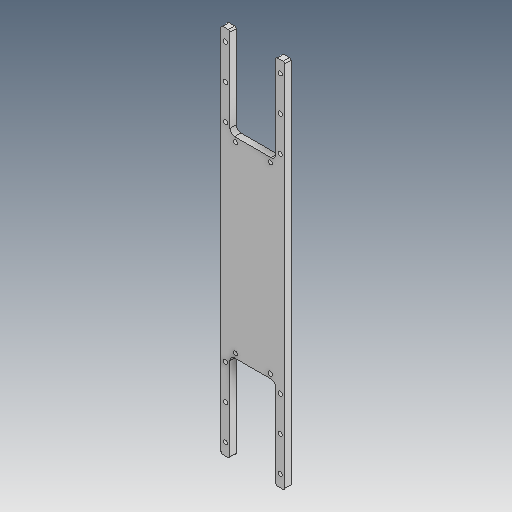
# Autodesk Inventor part: bar1
Saved by Autodesk Inventor 2020 (Build 240168000, 168)
## iProperties
Created: 2020-11-05
Part Number: bar1
Material: 일반
Document SubType Name: Sheet Metal
Designer: 이호석
Mass: 24.1768 g
Surface Area: 156.945 cm^2
Volume: 24.1768 cm^3
Density: 1 g/cm^3
Sheet Metal Rule: 기본값_mm
Appearance: 기본값
Author: 이호석
Autodesk Inventor part; units mm, degrees
ref_plane "YZ Plane" through (0, 0, 0) normal (1, 0, 0) x (0, 1, 0)
ref_plane "XZ Plane" through (0, 0, 0) normal (0, 1, 0) x (-1, 0, 0)
ref_plane "XY Plane" through (0, 0, 0) normal (0, 0, 1) x (1, 0, 0)
sketch "스케치1" plane through (0, 0, 0) normal (0, 0, 1) x (1, 0, 0)
  line L0 (-15, 14.5) -> (-11.5, 14.5)
  line L1 (-15, 14.5) -> (-20.1, 8.5)
  line L2 (-20.1, 8.5) -> (-20.1, -44.6)
  line L3 (-20.1, -44.6) -> (-15, -50.6)
  line L4 (-15, -50.6) -> (15, -50.6)
  line L5 (15, -50.6) -> (20.1, -44.6)
  line L6 (20.1, -44.6) -> (20.1, 8.5)
  line L7 (20.1, 8.5) -> (15, 14.5)
  line L8 (11.5, 14.5) -> (15, 14.5)
  arc A0 (14.5, 11.5) -> (11.5, 14.5) centre (11.5, 11.5) ccw
  line L9 (14.5, -42) -> (14.5, 11.5)
  arc A1 (11.5, -45) -> (14.5, -42) centre (11.5, -42) ccw
  line L10 (-11.5, -45) -> (11.5, -45)
  arc A2 (-14.5, -42) -> (-11.5, -45) centre (-11.5, -42) ccw
  line L11 (-14.5, 11.5) -> (-14.5, -42)
  arc A3 (-11.5, 14.5) -> (-14.5, 11.5) centre (-11.5, 11.5) ccw
  circle A4 centre (-17.3, 4) radius 1.35
  circle A5 centre (-17.3, -18) radius 1.35
  circle A6 centre (-11, -47.8) radius 1.35
  circle A7 centre (17.3, 4) radius 1.35
  circle A8 centre (17.3, -18) radius 1.35
  circle A9 centre (11, -47.8) radius 1.35
  circle A10 centre (-17.3, -40) radius 1.35
  circle A11 centre (17.3, -40) radius 1.35
  line L12 (15, -225.5) -> (11.5, -225.5)
  line L13 (15, -225.5) -> (20.1, -219.5)
  line L14 (20.1, -219.5) -> (20.1, -166.4)
  line L15 (20.1, -166.4) -> (15, -160.4)
  line L16 (15, -160.4) -> (-15, -160.4)
  line L17 (-15, -160.4) -> (-20.1, -166.4)
  line L18 (-20.1, -166.4) -> (-20.1, -219.5)
  line L19 (-20.1, -219.5) -> (-15, -225.5)
  line L20 (-11.5, -225.5) -> (-15, -225.5)
  arc A12 (-14.5, -222.5) -> (-11.5, -225.5) centre (-11.5, -222.5) ccw
  line L21 (-14.5, -169) -> (-14.5, -222.5)
  arc A13 (-11.5, -166) -> (-14.5, -169) centre (-11.5, -169) ccw
  line L22 (11.5, -166) -> (-11.5, -166)
  arc A14 (14.5, -169) -> (11.5, -166) centre (11.5, -169) ccw
  line L23 (14.5, -222.5) -> (14.5, -169)
  arc A15 (11.5, -225.5) -> (14.5, -222.5) centre (11.5, -222.5) ccw
  circle A16 centre (17.3, -215) radius 1.35
  circle A17 centre (17.3, -193) radius 1.35
  circle A18 centre (11, -163.2) radius 1.35
  circle A19 centre (-17.3, -215) radius 1.35
  circle A20 centre (-17.3, -193) radius 1.35
  circle A21 centre (-11, -163.2) radius 1.35
  circle A22 centre (17.3, -171) radius 1.35
  circle A23 centre (-17.3, -171) radius 1.35
  line L24 (20.1, -222.5) -> (20.1, 11.5)
  line L25 (-20.1, 11.5) -> (-20.1, -222.5)
  line L26 (14.5, -222.5) -> (14.5, -169)
  line L27 (11.5, -166) -> (-11.5, -166)
  line L28 (-14.5, -169) -> (-14.5, -222.5)
  arc A24 (14.5, -169) -> (11.5, -166) centre (11.5, -169) ccw
  arc A25 (-11.5, -166) -> (-14.5, -169) centre (-11.5, -169) ccw
  arc A26 (11.5, -45) -> (14.5, -42) centre (11.5, -42) ccw
  arc A27 (-14.5, -42) -> (-11.5, -45) centre (-11.5, -42) ccw
  line L29 (11.5, -45) -> (-11.5, -45)
  line L30 (-14.5, -42) -> (-14.5, 11.5)
  line L31 (14.5, 11.5) -> (14.5, -42)
  line L32 (20.1, 11.5) -> (14.5, 11.5)
  line L33 (-14.5, 11.5) -> (-20.1, 11.5)
  line L34 (-20.1, -222.5) -> (-14.5, -222.5)
  line L35 (14.5, -222.5) -> (20.1, -222.5)
  point P0 (0, 0)
  dimension "d0" = 3
  measures "d0" distance of L18.end L25.end
extrude "판1" add sketch "스케치1" along normal blind 4 contours L33 L11 A2 L10 A1 L9 L32 L7 L6 L5 L4 L3 L2 L1 | L1 L25 L33 | L3 L4 L5 L24 L15 L16 L17 L25 | L17 L16 L15 L14 L13 L35 L23 A14 L22 A13 L21 L34 L19 L18 | L19 L34 L25 | L7 L32 L24 | L24 L35 L13
fillet "모서리 라운드1" radius 1 8 edges at (14.5, -222.5, 2) (20.1, -222.5, 2) (-14.5, -222.5, 2) (-20.1, -222.5, 2) (-20.1, 11.5, 2) (-14.5, 11.5, 2) (14.5, 11.5, 2) (20.1, 11.5, 2)
equation "\"TransitionRadius\" = BendRadius"
equation "\"BendRadius\" = 4"
